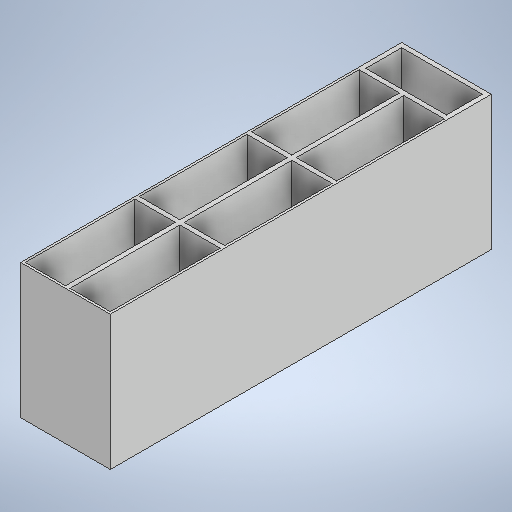
# Autodesk Inventor part: MoldsStore
Saved by Autodesk Inventor 2025.1 (Build 291241000, 241)
## iProperties
Created: 2025-02-10
Part Number: MoldsStore
Material: Generic
Document SubType Name: Modeling
Designer: yovan
Density: 1 g/cm^3
Appearance: Default
Author: yovan
Autodesk Inventor part; units mm, degrees
ref_plane "YZ Plane" through (0, 0, 0) normal (1, 0, 0) x (0, 1, 0)
ref_plane "XZ Plane" through (0, 0, 0) normal (0, 1, 0) x (-1, 0, 0)
ref_plane "XY Plane" through (0, 0, 0) normal (0, 0, 1) x (1, 0, 0)
sketch "Sketch2" plane through (0, 0, 0) normal (0, 1, 0) x (-1, 0, 0)
  line L0 (-400, 180) -> (-400, 1700)
  line L1 (-400, 1700) -> (0, 1700)
  line L2 (0, 1700) -> (0, 180)
  line L3 (-400, 200) -> (-400, 600)
  line L4 (0, 600) -> (0, 200)
  line L5 (0, 600) -> (0, 700)
  line L6 (-400, 700) -> (-400, 600)
  line L7 (-400, 700) -> (-400, 1100)
  line L8 (0, 1100) -> (0, 700)
  line L9 (0, 1100) -> (0, 1200)
  line L10 (-400, 1200) -> (-400, 1100)
  line L11 (-400, 1200) -> (-400, 1600)
  line L12 (0, 1600) -> (0, 1200)
  line L13 (0, 200) -> (0, 180)
  line L14 (0, 180) -> (-400, 180)
  line L15 (-400, 180) -> (-400, 200)
  line L16 (0, 700) -> (0, 680)
  line L17 (-400, 680) -> (-400, 700)
  line L18 (0, 1200) -> (0, 1180)
  line L19 (-400, 1180) -> (-400, 1200)
  line L20 (-390, 200) -> (-210, 200)
  line L21 (-190, 200) -> (-10, 200)
  line L22 (-10, 200) -> (-190, 200)
  line L23 (-210, 200) -> (-390, 200)
  line L24 (-210, 680) -> (-210, 200)
  line L25 (-190, 680) -> (-190, 200)
  line L26 (-390, 700) -> (-210, 700)
  line L27 (-190, 700) -> (-10, 700)
  line L28 (-10, 700) -> (-190, 700)
  line L29 (-210, 700) -> (-390, 700)
  line L30 (-10, 700) -> (-190, 700)
  line L31 (-210, 700) -> (-390, 700)
  line L32 (-10, 680) -> (-190, 680)
  line L33 (-210, 680) -> (-390, 680)
  line L34 (-10, 680) -> (-10, 200)
  line L35 (-390, 200) -> (-390, 680)
  line L36 (-210, 1690) -> (-210, 1200)
  line L37 (-210, 1180) -> (-210, 700)
  line L38 (-190, 1690) -> (-190, 1200)
  line L39 (-190, 1180) -> (-190, 700)
  line L40 (-390, 1200) -> (-210, 1200)
  line L41 (-190, 1200) -> (-10, 1200)
  line L42 (-10, 1200) -> (-190, 1200)
  line L43 (-210, 1200) -> (-390, 1200)
  line L44 (-10, 1200) -> (-190, 1200)
  line L45 (-210, 1200) -> (-390, 1200)
  line L46 (-10, 1180) -> (-190, 1180)
  line L47 (-210, 1180) -> (-390, 1180)
  line L48 (-10, 1690) -> (-10, 1200)
  line L49 (-10, 1180) -> (-10, 700)
  line L50 (-390, 700) -> (-390, 1180)
  line L51 (-390, 1200) -> (-390, 1690)
  line L52 (-390, 1690) -> (-210, 1690)
  line L53 (-190, 1690) -> (-10, 1690)
  point P0 (0, 0)
  dimension "d0" = 400
  dimension "d6" = 400
  dimension "d7" = 100
  dimension "d8" = 400
  dimension "d9" = 400
  dimension "d10" = 100
  dimension "d11" = 400
  dimension "d12" = 400
  dimension "d14" = 400
  dimension "d15" = 20
  dimension "d16" = 20
  dimension "d17" = 20
  dimension "d25" = 10
  constraints: 108 end point, 28 parallel, 12 horizontal, 12 perpendicular, 6 point on line
  measures "d0" distance of L0.end L1.end
  measures "d6" distance of L3.start L3.end
  measures "d7" distance of L5.end L5.start
  measures "d8" distance of L7.start L7.end
  measures "d9" distance of L10.start L9.end
  measures "d10" distance of L9.end L9.start
  measures "d11" distance of L11.end L12.start
  measures "d12" distance of L11.start L11.end
  measures "d14" distance of L2.end L0.start
  measures "d15" distance of L2.end L13.start
  measures "d16" distance of L16.start L16.end
  measures "d17" distance of L18.start L18.end
  measures "d25" distance between parallel lines of L48 L12
extrude "Extrusion1" add sketch "Sketch2" along normal blind 600
sketch "Sketch3" plane through (400, 0, 180) normal (0, 0, -1) x (-1, 0, 0)
  line L0 (0, 0) -> (400, 0)
  line L1 (400, 0) -> (400, 600)
  line L2 (400, 600) -> (0, 600)
  line L3 (0, 600) -> (0, 0)
  line L4 (20, 300) -> (380, 300)
  line L5 (200, 0) -> (200, 600)
  line L6 (0, 0) -> (20, 0)
  line L7 (20, 0) -> (20, 600)
  line L8 (20, 600) -> (0, 600)
  line L9 (0, 600) -> (0, 0)
  line L10 (400, 600) -> (380, 600)
  line L11 (380, 600) -> (380, 0)
  line L12 (380, 0) -> (400, 0)
  line L13 (400, 0) -> (400, 600)
  dimension "d20" = 20
  dimension "d21" = 20
  constraints: 28 end point, 6 parallel, 4 midpoint, 3 horizontal, 3 perpendicular, 2 point on line
  measures "d20" distance of L8.end L7.end
  measures "d21" distance of L12.end L11.end
extrude "Extrusion2" add sketch "Sketch3" along normal blind 200 contours L3 L2 L7 L0 | L11 L2 L1 L0
sketch "Sketch4" plane through (10, 0, 680) normal (1, 0, 0) x (0, 0, -1)
  line L0 (0, 0) -> (480, 0) projected
  line L1 (130, 0) -> (130, 250)
  line L2 (130, 0) -> (380, 0) construction
  line L3 (130, 250) -> (140, 250)
  line L4 (140, 250) -> (140, 0)
  line L5 (130, 0) -> (140, 0)
  point P0 (680, 0)
  dimension "d26" = 250
  dimension "d27" = 90
  dimension "d28" = 10
  constraints: 10 end point, 3 perpendicular, 2 point on line, 2 vertical, 1 horizontal
  measures "d26" distance of L1.start L1.end
  measures "d27" angle of L2 L1
  measures "d28" distance of L1.end L3.end
extrude "Extrusion3" add sketch "Sketch4" along normal blind 35
sketch "Sketch5" plane through (10, 0, 1180) normal (1, 0, 0) x (0, 0, -1)
  line L0 (0, 0) -> (480, 0) projected
  line L1 (130, 0) -> (130, 250)
  line L2 (130, 0) -> (380, 0) construction
  line L3 (130, 250) -> (140, 250)
  line L4 (140, 250) -> (140, 0)
  line L5 (140, 0) -> (130, 0)
  line L6 (-510, 0) -> (-20, 0) projected
  line L7 (-370, 0) -> (-370, 250)
  line L8 (-370, 0) -> (-120, 0) construction
  line L9 (-370, 250) -> (-360, 250)
  line L10 (-360, 250) -> (-360, 0)
  line L11 (-360, 0) -> (-370, 0)
  point P0 (1180, 0)
  point P1 (-360, 0)
  dimension "d31" = 250
  dimension "d32" = 90
  dimension "d33" = 10
  dimension "d34" = 250
  dimension "d35" = 90
  dimension "d36" = 10
  dimension "d37" = 90
  dimension "d38" = 90
  constraints: 20 end point, 7 perpendicular, 2 horizontal, 2 point on line, 2 vertical
  measures "d31" distance of L1.start L1.end
  measures "d32" angle of L2 L1
  measures "d33" distance of L1.end L3.end
  measures "d34" distance of L7.start L7.end
  measures "d35" angle of L8 L7
  measures "d36" distance of L7.end L9.end
  measures "d37" angle of L7 L9
  measures "d38" angle of L9 L10
extrude "Extrusion4" add sketch "Sketch5" along normal blind 35
sketch "Sketch7" plane through (20, 0, 180) normal (1, 0, 0) x (0, 0, -1)
  line L0 (-1520, 0) -> (200, 0) projected
  line L1 (200, 0) -> (160, 0)
  line L2 (160, 0) -> (160, 600)
  line L3 (160, 600) -> (200, 600)
  line L4 (200, 600) -> (200, 0)
  point P0 (180, 0)
  point P1 (160, 0)
  dimension "d49" = 40
  dimension "d50" = 600
  constraints: 8 end point, 2 parallel, 1 horizontal, 1 perpendicular
  measures "d49" distance of L2.end L3.end
  measures "d50" distance of L1.end L2.end
extrude "Extrusion6" add sketch "Sketch7" along normal blind 370
sketch "Sketch8" plane through (390, 0, 200) normal (-1, 0, 0) x (0, 0, 1)
  line L0 (1500, 0) -> (-220, 0) projected
  line L1 (350, 0) -> (340, 0)
  line L2 (340, 0) -> (340, 250)
  line L3 (340, 250) -> (350, 250)
  line L4 (350, 250) -> (350, 0)
  line L5 (850, 0) -> (840, 0)
  line L6 (840, 0) -> (840, 250)
  line L7 (840, 250) -> (850, 250)
  line L8 (850, 250) -> (850, 0)
  line L9 (1350, 0) -> (1340, 0)
  line L10 (1340, 0) -> (1340, 250)
  line L11 (1340, 250) -> (1350, 250)
  line L12 (1350, 250) -> (1350, 0)
  point P0 (-200, 0)
  dimension "d53" = 10
  dimension "d54" = 250
  dimension "d55" = 10
  dimension "d56" = 250
  dimension "d57" = 10
  dimension "d58" = 250
  constraints: 24 end point, 6 parallel, 3 horizontal, 3 perpendicular, 3 point on line
  measures "d53" distance of L2.end L3.end
  measures "d54" distance of L1.end L2.end
  measures "d55" distance of L6.end L7.end
  measures "d56" distance of L5.end L6.end
  measures "d57" distance of L10.end L11.end
  measures "d58" distance of L9.end L10.end
extrude "Extrusion7" add sketch "Sketch8" along normal blind 35
sketch "Sketch9" plane through (400, 0, -20) normal (0, 0, -1) x (-1, 0, 0)
  line L0 (400, 600) -> (0, 600) projected
  line L1 (400, 600) -> (0, 600)
  line L2 (0, 600) -> (0, 0)
  line L3 (0, 0) -> (400, 0)
  line L4 (400, 0) -> (400, 600)
  point P0 (400, 0)
  constraints: 8 end point, 2 parallel, 1 horizontal, 1 perpendicular
extrude "Extrusion8" cut sketch "Sketch9" against normal blind 20
body "Solid1"
